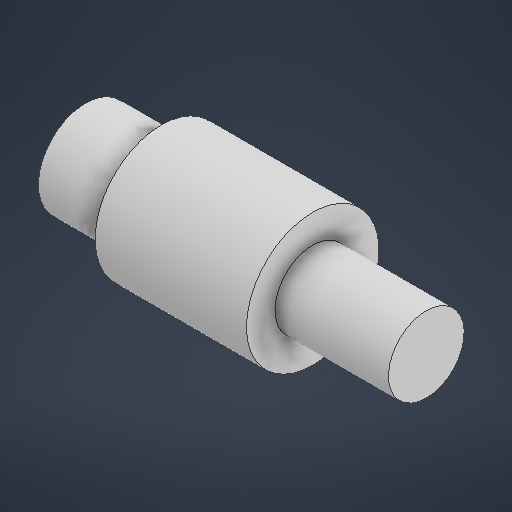
# Autodesk Inventor part: Part12
Saved by Autodesk Inventor 2026 (Build 300175050, 175E)
## iProperties
Created: 2026-03-26
Part Number: Part12
Material: Generic
Document SubType Name: Modeling
Designer: Administrator
Density: 1 g/cm^3
Appearance: Default
Author: Administrator
Autodesk Inventor part; units mm, degrees
ref_plane "YZ Plane" through (0, 0, 0) normal (1, 0, 0) x (0, 1, 0)
ref_plane "XZ Plane" through (0, 0, 0) normal (0, 1, 0) x (-1, 0, 0)
ref_plane "XY Plane" through (0, 0, 0) normal (0, 0, 1) x (1, 0, 0)
sketch "Sketch1" plane through (0, 0, 0) normal (0, 0, 1) x (1, 0, 0)
  line L0 (0, 0) -> (90, 0)
  line L1 (90, 0) -> (90, 10)
  line L2 (90, 10) -> (60, 10)
  line L3 (60, 10) -> (60, 17.5)
  line L4 (60, 17.5) -> (20, 17.5)
  line L5 (20, 17.5) -> (20, 12.5)
  line L6 (20, 12.5) -> (0, 12.5)
  line L7 (0, 12.5) -> (0, 0)
  dimension "d0" = 90
  dimension "d1" = 40
  dimension "d2" = 20
  dimension "d3" = 20
  dimension "d4" = 35
  dimension "d5" = 25
  constraints: 16 end point, 6 perpendicular, 1 horizontal, 1 vertical
  measures "d0" distance of L0.start L0.end
  measures "d1" distance of L3.end L4.end
  measures "d2" distance of L5.end L6.end
  measures "d3" diameter of L2 L0
  measures "d4" diameter of L4 L0
  measures "d5" diameter of L6 L0
revolve "Revolution1" add sketch "Sketch1" angle 360 mid plane about axis through (0, 0, 0) along (1, 0, 0)
body "Solid1"
